Autodesk Inventor part; units mm, degrees
(part 2 of 2)
  spline S155 degree 2 poles (-17.7724, 9.7369) (-16.6749, 9.7369) (-15.9843, 9.0875) knots 0 0 0 1 1 1
  spline S156 degree 2 poles (-15.9843, 9.0875) (-15.5773, 8.7033) (-15.3715, 7.9853) knots 0 0 0 1 1 1
  line L514 (-15.3715, 7.9853) -> (-16.5697, 7.6972)
  spline S157 degree 2 poles (-16.5697, 7.6972) (-16.6749, 8.1637) (-17.3517, 8.7033) (-17.8319, 8.7033) knots 0 0 0 1 2 2 2
  spline S158 degree 2 poles (-17.8319, 8.7033) (-18.4996, 8.7033) (-19.3319, 7.7475) (-19.3319, 6.6728) knots 0 0 0 1 2 2 2
  spline S159 degree 2 poles (-19.3319, 6.6728) (-19.3319, 5.5341) (-18.5133, 4.5692) (-17.8593, 4.5692) knots 0 0 0 1 2 2 2
  spline S160 degree 2 poles (-17.8593, 4.5692) (-17.3746, 4.5692) (-16.6794, 5.1865) (-16.5285, 5.8451) knots 0 0 0 1 2 2 2
  line L515 (-49.6634, -5.806) -> (-50.9805, -5.806)
  line L516 (-50.9805, -5.806) -> (-51.5018, -4.4432)
  line L517 (-51.5018, -4.4432) -> (-53.8982, -4.4432)
  line L518 (-53.8982, -4.4432) -> (-54.3967, -5.806)
  line L519 (-54.3967, -5.806) -> (-55.6817, -5.806)
  line L520 (-55.6817, -5.806) -> (-53.3494, 0.194)
  line L521 (-53.3494, 0.194) -> (-52.0598, 0.194)
  line L522 (-52.0598, 0.194) -> (-49.6634, -5.806)
  line L523 (-51.8906, -3.4279) -> (-52.7183, -1.2054)
  line L524 (-52.7183, -1.2054) -> (-53.5323, -3.4279)
  line L525 (-53.5323, -3.4279) -> (-51.8906, -3.4279)
  line L526 (-49.0049, -5.806) -> (-49.0049, 0.194)
  line L527 (-49.0049, 0.194) -> (-47.8296, 0.194)
  line L528 (-47.8296, 0.194) -> (-45.3647, -3.8304)
  line L529 (-45.3647, -3.8304) -> (-45.3647, 0.194)
  line L530 (-45.3647, 0.194) -> (-44.2442, 0.194)
  line L531 (-44.2442, 0.194) -> (-44.2442, -5.806)
  line L532 (-44.2442, -5.806) -> (-45.4561, -5.806)
  line L533 (-45.4561, -5.806) -> (-47.8845, -1.8685)
  line L534 (-47.8845, -1.8685) -> (-47.8845, -5.806)
  line L535 (-47.8845, -5.806) -> (-49.0049, -5.806)
  line L536 (-41.6101, -5.806) -> (-41.6101, -0.8212)
  line L537 (-41.6101, -0.8212) -> (-43.389, -0.8212)
  line L538 (-43.389, -0.8212) -> (-43.389, 0.194)
  line L539 (-43.389, 0.194) -> (-38.6238, 0.194)
  line L540 (-38.6238, 0.194) -> (-38.6238, -0.8212)
  line L541 (-38.6238, -0.8212) -> (-40.3982, -0.8212)
  line L542 (-40.3982, -0.8212) -> (-40.3982, -5.806)
  line L543 (-40.3982, -5.806) -> (-41.6101, -5.806)
  line L544 (-37.8372, -5.806) -> (-37.8372, 0.194)
  line L545 (-37.8372, 0.194) -> (-33.3875, 0.194)
  line L546 (-33.3875, 0.194) -> (-33.3875, -0.8212)
  line L547 (-33.3875, -0.8212) -> (-36.6253, -0.8212)
  line L548 (-36.6253, -0.8212) -> (-36.6253, -2.152)
  line L549 (-36.6253, -2.152) -> (-33.6116, -2.152)
  line L550 (-33.6116, -2.152) -> (-33.6116, -3.1673)
  line L551 (-33.6116, -3.1673) -> (-36.6253, -3.1673)
  line L552 (-36.6253, -3.1673) -> (-36.6253, -4.7907)
  line L553 (-36.6253, -4.7907) -> (-33.2732, -4.7907)
  line L554 (-33.2732, -4.7907) -> (-33.2732, -5.806)
  line L555 (-33.2732, -5.806) -> (-37.8372, -5.806)
  line L556 (-32.2351, -5.806) -> (-32.2351, 0.194)
  line L557 (-32.2351, 0.194) -> (-31.0598, 0.194)
  line L558 (-31.0598, 0.194) -> (-28.5948, -3.8304)
  line L559 (-28.5948, -3.8304) -> (-28.5948, 0.194)
  line L560 (-28.5948, 0.194) -> (-27.4744, 0.194)
  line L561 (-27.4744, 0.194) -> (-27.4744, -5.806)
  line L562 (-27.4744, -5.806) -> (-28.6863, -5.806)
  line L563 (-28.6863, -5.806) -> (-31.1147, -1.8685)
  line L564 (-31.1147, -1.8685) -> (-31.1147, -5.806)
  line L565 (-31.1147, -5.806) -> (-32.2351, -5.806)
  line L566 (-26.1802, -5.806) -> (-26.1802, 0.194)
  line L567 (-26.1802, 0.194) -> (-25.0049, 0.194)
  line L568 (-25.0049, 0.194) -> (-22.54, -3.8304)
  line L569 (-22.54, -3.8304) -> (-22.54, 0.194)
  line L570 (-22.54, 0.194) -> (-21.4195, 0.194)
  line L571 (-21.4195, 0.194) -> (-21.4195, -5.806)
  line L572 (-21.4195, -5.806) -> (-22.6314, -5.806)
  line L573 (-22.6314, -5.806) -> (-25.0598, -1.8685)
  line L574 (-25.0598, -1.8685) -> (-25.0598, -5.806)
  line L575 (-25.0598, -5.806) -> (-26.1802, -5.806)
  line L576 (-14.729, -5.806) -> (-16.0461, -5.806)
  line L577 (-16.0461, -5.806) -> (-16.5674, -4.4432)
  line L578 (-16.5674, -4.4432) -> (-18.9637, -4.4432)
  line L579 (-18.9637, -4.4432) -> (-19.4622, -5.806)
  line L580 (-19.4622, -5.806) -> (-20.7473, -5.806)
  line L581 (-20.7473, -5.806) -> (-18.415, 0.194)
  line L582 (-18.415, 0.194) -> (-17.1253, 0.194)
  line L583 (-17.1253, 0.194) -> (-14.729, -5.806)
  line L584 (-16.9561, -3.4279) -> (-17.7839, -1.2054)
  line L585 (-17.7839, -1.2054) -> (-18.5979, -3.4279)
  line L586 (-18.5979, -3.4279) -> (-16.9561, -3.4279)
  spline S161 degree 2 poles (-54.3121, -9.2253) (-53.4386, -9.2253) (-52.9493, -9.8473) knots 0 0 0 1 1 1
  spline S162 degree 2 poles (-52.9493, -9.8473) (-52.3639, -10.5836) (-52.3639, -12.2893) knots 0 0 0 1 1 1
  spline S163 degree 2 poles (-52.3639, -12.2893) (-52.3639, -13.9906) (-52.9538, -14.736) knots 0 0 0 1 1 1
  spline S164 degree 2 poles (-52.9538, -14.736) (-53.4386, -15.3488) (-54.3121, -15.3488) knots 0 0 0 1 1 1
  spline S165 degree 2 poles (-54.3121, -15.3488) (-55.1901, -15.3488) (-56.2602, -14.0043) (-56.2602, -12.2756) knots 0 0 0 1 2 2 2
  spline S166 degree 2 poles (-56.2602, -12.2756) (-56.2602, -10.5836) (-55.6703, -9.8381) knots 0 0 0 1 1 1
  spline S167 degree 2 poles (-55.6703, -9.8381) (-55.1855, -9.2253) (-54.3121, -9.2253) knots 0 0 0 1 1 1
  spline S168 degree 2 poles (-54.3121, -10.1811) (-54.5224, -10.1811) (-54.8471, -10.4464) (-54.9386, -10.7893) knots 0 0 0 1 2 2 2
  spline S169 degree 2 poles (-54.9386, -10.7893) (-55.0575, -11.2329) (-55.0575, -12.2893) knots 0 0 0 1 1 1
  spline S170 degree 2 poles (-55.0575, -12.2893) (-55.0575, -13.3412) (-54.8425, -14.1323) (-54.5224, -14.393) (-54.3121, -14.393) knots 0 0 0 1 2 3 3 3
  spline S171 degree 2 poles (-54.3121, -14.393) (-54.1017, -14.393) (-53.777, -14.1278) (-53.6855, -13.7848) knots 0 0 0 1 2 2 2
  spline S172 degree 2 poles (-53.6855, -13.7848) (-53.5666, -13.3412) (-53.5666, -12.2893) knots 0 0 0 1 1 1
  spline S173 degree 2 poles (-53.5666, -12.2893) (-53.5666, -11.2329) (-53.7816, -10.4464) (-54.1017, -10.1811) (-54.3121, -10.1811) knots 0 0 0 1 2 3 3 3
  line L587 (-51.3532, -15.2482) -> (-51.3532, -14.0957)
  line L588 (-51.3532, -14.0957) -> (-50.2008, -14.0957)
  line L589 (-50.2008, -14.0957) -> (-50.2008, -15.2482)
  line L590 (-50.2008, -15.2482) -> (-51.3532, -15.2482)
  spline S174 degree 2 poles (-48.2846, -12.0104) (-48.7282, -11.8229) (-49.1352, -11.1643) (-49.1352, -10.7711) knots 0 0 0 1 2 2 2
  spline S175 degree 2 poles (-49.1352, -10.7711) (-49.1352, -10.0988) (-48.1977, -9.2253) (-47.3334, -9.2253) knots 0 0 0 1 2 2 2
  spline S176 degree 2 poles (-47.3334, -9.2253) (-46.4782, -9.2253) (-45.5316, -10.0988) (-45.5316, -10.7711) knots 0 0 0 1 2 2 2
  spline S177 degree 2 poles (-45.5316, -10.7711) (-45.5316, -11.1872) (-45.966, -11.8366) (-46.3593, -12.0104) knots 0 0 0 1 2 2 2
  spline S178 degree 2 poles (-46.3593, -12.0104) (-45.8608, -12.2116) (-45.3395, -12.9799) (-45.3395, -13.4829) knots 0 0 0 1 2 2 2
  spline S179 degree 2 poles (-45.3395, -13.4829) (-45.3395, -14.3153) (-46.4005, -15.3534) (-47.2785, -15.3534) knots 0 0 0 1 2 2 2
  spline S180 degree 2 poles (-47.2785, -15.3534) (-48.0971, -15.3534) (-48.6413, -14.9235) knots 0 0 0 1 1 1
  spline S181 degree 2 poles (-48.6413, -14.9235) (-49.2861, -14.4159) (-49.2861, -13.5332) knots 0 0 0 1 1 1
  spline S182 degree 2 poles (-49.2861, -13.5332) (-49.2861, -13.0439) (-48.8014, -12.2299) (-48.2846, -12.0104) knots 0 0 0 1 2 2 2
  spline S183 degree 2 poles (-48.152, -13.4235) (-48.152, -13.8991) (-47.6672, -14.4296) (-47.3014, -14.4296) knots 0 0 0 1 2 2 2
  spline S184 degree 2 poles (-47.3014, -14.4296) (-46.9447, -14.4296) (-46.4782, -13.9174) (-46.4782, -13.4326) knots 0 0 0 1 2 2 2
  spline S185 degree 2 poles (-46.4782, -13.4326) (-46.4782, -13.0119) (-46.9538, -12.4997) (-47.3151, -12.4997) knots 0 0 0 1 2 2 2
  spline S186 degree 2 poles (-47.3151, -12.4997) (-47.7404, -12.4997) (-48.152, -13.0805) (-48.152, -13.4235) knots 0 0 0 1 2 2 2
  spline S187 degree 2 poles (-48.0468, -10.8534) (-48.0468, -11.1964) (-47.6581, -11.5805) (-47.3334, -11.5805) knots 0 0 0 1 2 2 2
  spline S188 degree 2 poles (-47.3334, -11.5805) (-47.0041, -11.5805) (-46.6108, -11.1918) (-46.6108, -10.8488) knots 0 0 0 1 2 2 2
  spline S189 degree 2 poles (-46.6108, -10.8488) (-46.6108, -10.5287) (-46.9996, -10.14) (-47.3197, -10.14) knots 0 0 0 1 2 2 2
  spline S190 degree 2 poles (-47.3197, -10.14) (-47.6535, -10.14) (-48.0468, -10.5332) (-48.0468, -10.8534) knots 0 0 0 1 2 2 2
  line L591 (-42.1657, -13.6476) -> (-42.1657, -12.4951)
  line L592 (-42.1657, -12.4951) -> (-39.9066, -12.4951)
  line L593 (-39.9066, -12.4951) -> (-39.9066, -13.6476)
  line L594 (-39.9066, -13.6476) -> (-42.1657, -13.6476)
  line L595 (-33.2663, -10.7162) -> (-34.3776, -10.8397)
  spline S191 degree 2 poles (-34.3776, -10.8397) (-34.4188, -10.4967) (-34.7618, -10.172) (-35.0361, -10.172) knots 0 0 0 1 2 2 2
  spline S192 degree 2 poles (-35.0361, -10.172) (-35.402, -10.172) (-35.905, -10.8259) (-35.9691, -11.8595) knots 0 0 0 1 2 2 2
  spline S193 degree 2 poles (-35.9691, -11.8595) (-35.5438, -11.3518) (-34.9035, -11.3518) knots 0 0 0 1 1 1
  spline S194 degree 2 poles (-34.9035, -11.3518) (-34.1855, -11.3518) (-33.1566, -12.4494) (-33.1566, -13.3137) knots 0 0 0 1 2 2 2
  spline S195 degree 2 poles (-33.1566, -13.3137) (-33.1566, -14.2375) (-34.2358, -15.3488) (-35.0819, -15.3488) knots 0 0 0 1 2 2 2
  spline S196 degree 2 poles (-35.0819, -15.3488) (-35.9919, -15.3488) (-37.1627, -13.9357) (-37.1627, -12.3305) knots 0 0 0 1 2 2 2
  spline S197 degree 2 poles (-37.1627, -12.3305) (-37.1627, -10.6796) (-35.9416, -9.2253) (-34.9675, -9.2253) knots 0 0 0 1 2 2 2
  spline S198 degree 2 poles (-34.9675, -9.2253) (-34.2861, -9.2253) (-33.3898, -9.989) (-33.2663, -10.7162) knots 0 0 0 1 2 2 2
  spline S199 degree 2 poles (-35.873, -13.2223) (-35.873, -13.7848) (-35.3563, -14.393) (-35.027, -14.393) knots 0 0 0 1 2 2 2
  spline S200 degree 2 poles (-35.027, -14.393) (-34.7069, -14.393) (-34.2816, -13.8945) (-34.2816, -13.3275) knots 0 0 0 1 2 2 2
  spline S201 degree 2 poles (-34.2816, -13.3275) (-34.2816, -12.7421) (-34.7389, -12.1979) (-35.0819, -12.1979) knots 0 0 0 1 2 2 2
  spline S202 degree 2 poles (-35.0819, -12.1979) (-35.4157, -12.1979) (-35.873, -12.7192) (-35.873, -13.2223) knots 0 0 0 1 2 2 2
  line L596 (-27.1291, -13.0485) -> (-27.1291, -12.0332)
  line L597 (-27.1291, -12.0332) -> (-24.5179, -12.0332)
  line L598 (-24.5179, -12.0332) -> (-24.5179, -14.4204)
  spline S203 degree 2 poles (-24.5179, -14.4204) (-24.8974, -14.7909) (-26.3425, -15.3488) (-27.0834, -15.3488) knots 0 0 0 1 2 2 2
  spline S204 degree 2 poles (-27.0834, -15.3488) (-28.0255, -15.3488) (-29.4249, -14.5576) (-30.1291, -13.0897) (-30.1291, -12.2299) knots 0 0 0 1 2 3 3 3
  spline S205 degree 2 poles (-30.1291, -12.2299) (-30.1291, -11.2924) (-29.3425, -9.8336) (-28.588, -9.4448) knots 0 0 0 1 2 2 2
  spline S206 degree 2 poles (-28.588, -9.4448) (-28.0072, -9.1476) (-27.1474, -9.1476) knots 0 0 0 1 1 1
  spline S207 degree 2 poles (-27.1474, -9.1476) (-26.0316, -9.1476) (-24.7739, -10.0851) (-24.5956, -10.9128) knots 0 0 0 1 2 2 2
  line L599 (-24.5956, -10.9128) -> (-25.7983, -11.1369)
  spline S208 degree 2 poles (-25.7983, -11.1369) (-25.9264, -10.6933) (-26.6261, -10.1811) (-27.1474, -10.1811) knots 0 0 0 1 2 2 2
  spline S209 degree 2 poles (-27.1474, -10.1811) (-27.9432, -10.1811) (-28.8807, -11.1872) (-28.8807, -12.1796) knots 0 0 0 1 2 2 2
  spline S210 degree 2 poles (-28.8807, -12.1796) (-28.8807, -13.2451) (-27.9294, -14.3153) (-27.1611, -14.3153) knots 0 0 0 1 2 2 2
  spline S211 degree 2 poles (-27.1611, -14.3153) (-26.7816, -14.3153) (-26.0179, -14.018) (-25.7435, -13.8076) knots 0 0 0 1 2 2 2
  line L600 (-25.7435, -13.8076) -> (-25.7435, -13.0485)
  line L601 (-25.7435, -13.0485) -> (-27.1291, -13.0485)
  line L602 (-23.3974, -15.2482) -> (-23.3974, -9.2482)
  line L603 (-23.3974, -9.2482) -> (-22.1855, -9.2482)
  line L604 (-22.1855, -9.2482) -> (-22.1855, -11.6079)
  line L605 (-22.1855, -11.6079) -> (-19.8121, -11.6079)
  line L606 (-19.8121, -11.6079) -> (-19.8121, -9.2482)
  line L607 (-19.8121, -9.2482) -> (-18.6002, -9.2482)
  line L608 (-18.6002, -9.2482) -> (-18.6002, -15.2482)
  line L609 (-18.6002, -15.2482) -> (-19.8121, -15.2482)
  line L610 (-19.8121, -15.2482) -> (-19.8121, -12.6232)
  line L611 (-19.8121, -12.6232) -> (-22.1855, -12.6232)
  line L612 (-22.1855, -12.6232) -> (-22.1855, -15.2482)
  line L613 (-22.1855, -15.2482) -> (-23.3974, -15.2482)
  line L614 (-17.8182, -15.2482) -> (-17.8182, -14.3427)
  line L615 (-17.8182, -14.3427) -> (-16.1901, -12.4814)
  spline S212 degree 2 poles (-16.1901, -12.4814) (-15.7877, -12.0241) (-15.5956, -11.832) knots 0 0 0 1 1 1
  spline S213 degree 2 poles (-15.5956, -11.832) (-15.7968, -11.8412) (-16.1215, -11.8457) knots 0 0 0 1 1 1
  line L616 (-16.1215, -11.8457) -> (-17.6581, -11.8549)
  line L617 (-17.6581, -11.8549) -> (-17.6581, -10.8991)
  line L618 (-17.6581, -10.8991) -> (-14.0636, -10.8991)
  line L619 (-14.0636, -10.8991) -> (-14.0636, -11.7177)
  line L620 (-14.0636, -11.7177) -> (-15.7282, -13.6293)
  line L621 (-15.7282, -13.6293) -> (-16.3136, -14.2604)
  spline S214 degree 2 poles (-16.3136, -14.2604) (-15.8334, -14.2375) (-15.7191, -14.2375) knots 0 0 0 1 1 1
  line L622 (-15.7191, -14.2375) -> (-13.9355, -14.2375)
  line L623 (-13.9355, -14.2375) -> (-13.9355, -15.2482)
  line L624 (-13.9355, -15.2482) -> (-17.8182, -15.2482)
  point P0 (0, 0)
  point P1 (25.9751, 2.0414)
  point P2 (37.5026, -3.8332)
  point P3 (37.924, -3.5043)
  point P4 (4.0294, -3.8332)
  point P5 (4.4507, -3.5043)
  point P6 (15.5407, -2.5986)
  point P7 (15.7392, -3.0593)
  point P8 (16.6191, -3.377)
  point P9 (18.2891, -3.8412)
  point P10 (19.1855, -4.6079)
  point P11 (14.4924, -7.7376)
  point P12 (16.4574, -5.2246)
  point P13 (14.4261, -4.4189)
  point P14 (13.8216, -2.9208)
  point P15 (5.1748, -0.8882)
  point P16 (6.0801, -1.6568)
  point P17 (6.4415, -2.9105)
  point P18 (5.1439, -4.8431)
  point P19 (41.6612, -1.6349)
  point P20 (42.7124, -4.4216)
  point P21 (44.1315, -6.8305)
  point P22 (45.4498, -5.418)
  point P23 (44.1022, -8.2594)
  point P24 (38.648, -0.8882)
  point P25 (39.5534, -1.6568)
  point P26 (39.9147, -2.9105)
  point P27 (55.7356, 4.9479)
  point P28 (56.3776, 6.4053)
  point P29 (55.9895, 7.5379)
  point P30 (54.8238, 8.2337)
  point P31 (56.1696, 9.8923)
  point P32 (55.8631, 10.9329)
  point P33 (53.8741, 10.4462)
  point P34 (26.4423, 5.6608)
  point P35 (26.4247, 11.9349)
  point P36 (23.9993, 5.2556)
  point P37 (26.413, 4.2318)
  point P38 (3.5164, 4.9479)
  point P39 (4.1585, 6.4053)
  point P40 (3.7703, 7.5379)
  point P41 (2.6047, 8.2337)
  point P42 (3.9504, 9.8923)
  point P43 (3.6439, 10.9329)
  point P44 (0.9228, 10.5005)
  point P45 (1.6549, 10.4462)
  point P46 (1.1473, 7.5332)
  point P47 (2.0452, 5.9728)
  dimension "d0" = 6.9444
  dimension "d1" = 6.381
  constraints: 310 end point, 299 other
  measures "d0" distance between parallel lines of L219 L453
  measures "d1" distance between parallel lines of L453 L26
extrude "Extrusion1" add sketch "Sketch1" along normal blind 1
body "Solid1"
